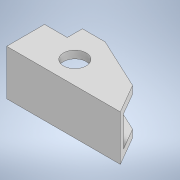
# Autodesk Inventor part: GuideBlock
Saved by Autodesk Inventor 2022.2 (Build 262287030, 287C)
## iProperties
Created: 2023-02-08
Part Number: GuideBlock
Material: Generic
Document SubType Name: Modeling
Designer: jak27277
Density: 1 g/cm^3
Appearance: Default
Author: jak27277
Autodesk Inventor part; units mm, degrees
ref_plane "YZ Plane" through (0, 0, 0) normal (1, 0, 0) x (0, 1, 0)
ref_plane "XZ Plane" through (0, 0, 0) normal (0, 1, 0) x (-1, 0, 0)
ref_plane "XY Plane" through (0, 0, 0) normal (0, 0, 1) x (1, 0, 0)
sketch "Sketch1" plane through (0, 0, 0) normal (0, 1, 0) x (-1, 0, 0)
  circle A0 centre (0, 0) radius 9.525
  line L0 (38.1, -12.7) -> (19.05, -12.7)
  line L1 (19.05, -12.7) -> (19.05, -25.4)
  line L2 (19.05, -25.4) -> (0, -25.4)
  line L3 (0, -25.4) -> (-43.0867, -5.3083)
  line L4 (-43.0867, -5.3083) -> (-57.15, 19.05)
  line L5 (-57.15, 19.05) -> (38.1, 19.05)
  line L6 (38.1, 19.05) -> (38.1, -12.7)
  dimension "d0" = 31.75
  dimension "d1" = 44.45
  dimension "d2" = 38.1
  dimension "d3" = 19.05
  dimension "d4" = 95.25
  dimension "d5" = 60
  dimension "d6" = 25
  dimension "d7" = 38.1
  dimension "d8" = 19.05
  dimension "d9" = 19.05
  constraints: 14 end point, 3 perpendicular, 2 horizontal, 1 centre point, 1 coincident
  measures "d0" distance of L5.end L0.start
  measures "d1" distance between parallel lines of L2 L5
  measures "d2" distance from line of L2.end L6
  measures "d3" distance of L0.start L0.end
  measures "d4" distance of L4.end L5.end
  measures "d5" angle of L5 L4
  measures "d6" angle of L2 L3
  measures "d7" distance from line of L6 point (0, 0)
  measures "d8" distance from line of L5 point (0, 0)
  measures "d9" diameter of A0
extrude "Extrusion1" add sketch "Sketch1" along normal blind 38.1
shell "Shell1" thickness 6.35 removed faces 6 at (-25.4, 12.7, -12.7) at (-19.05, 12.7, -21.1667) at (52.4622, 12.7, 10.9306) at (-6.35, 12.7, -25.4) at (28.7245, 12.7, -12.0056) at (-9.4017, 25.4, -1.5279)
body "Solid1"
